Autodesk Fusion 360 part; units mm, degrees
note: some values were not read from the file. Set by a fixed rule: which sketch regions a step uses.
(part 4 of 4)
sketch "Sketch12" plane through (0, 0, 0) normal (0, 0, -1) x (1, 0, 0)
  arc A0 (214.104, -171.958) -> (214.104, -165.862) centre (214.104, -168.91) ccw
  line L0 (214.104, -171.958) -> (197.3761, -171.958)
  arc A1 (197.3761, -165.862) -> (197.3761, -171.958) centre (197.3761, -168.91) ccw
  line L1 (197.3761, -165.862) -> (214.104, -165.862)
  arc A2 (216.662, -132.8241) -> (222.758, -132.8241) centre (219.71, -132.8241) ccw
  line L2 (216.662, -132.8241) -> (216.662, -113.5562)
  arc A3 (222.758, -113.5562) -> (216.662, -113.5562) centre (219.71, -113.5562) ccw
  line L3 (222.758, -113.5562) -> (222.758, -132.8241)
  arc A4 (247.142, -132.8241) -> (253.238, -132.8241) centre (250.19, -132.8241) ccw
  line L4 (247.142, -132.8241) -> (247.142, -113.5562)
  arc A5 (253.238, -113.5562) -> (247.142, -113.5562) centre (250.19, -113.5562) ccw
  line L5 (253.238, -113.5562) -> (253.238, -132.8241)
  arc A6 (253.238, -144.0361) -> (247.142, -144.0361) centre (250.19, -144.0361) ccw
  line L6 (253.238, -144.0361) -> (253.238, -163.304)
  arc A7 (247.142, -163.304) -> (253.238, -163.304) centre (250.19, -163.304) ccw
  line L7 (247.142, -163.304) -> (247.142, -144.0361)
  line L8 (275.082, -163.304) -> (275.082, -144.0361)
  arc A8 (281.178, -144.0361) -> (275.082, -144.0361) centre (278.13, -144.0361) ccw
  line L9 (281.178, -144.0361) -> (281.178, -163.304)
  arc A9 (275.082, -163.304) -> (281.178, -163.304) centre (278.13, -163.304) ccw
  arc A10 (255.796, -104.9022) -> (255.796, -110.9982) centre (255.796, -107.9502) ccw
  line L10 (255.796, -104.9022) -> (272.5239, -104.9022)
  arc A11 (272.5239, -110.9982) -> (272.5239, -104.9022) centre (272.5239, -107.9502) ccw
  line L11 (272.5239, -110.9982) -> (255.796, -110.9982)
  arc A12 (188.722, -132.824) -> (194.818, -132.8241) centre (191.77, -132.824) ccw
  line L12 (188.722, -132.824) -> (188.722, -113.5562)
  arc A13 (194.818, -113.5562) -> (188.722, -113.5562) centre (191.77, -113.5562) ccw
  line L13 (194.818, -113.5562) -> (194.818, -132.8241)
  arc A14 (194.818, -144.0361) -> (188.722, -144.0361) centre (191.77, -144.0361) ccw
  line L14 (194.818, -144.0361) -> (194.818, -163.304)
  arc A15 (188.722, -163.304) -> (194.818, -163.304) centre (191.77, -163.304) ccw
  line L15 (188.722, -163.304) -> (188.722, -144.0361)
  arc A16 (214.104, -141.4781) -> (214.104, -135.3821) centre (214.104, -138.4301) ccw
  line L16 (214.104, -141.4781) -> (197.3761, -141.4781)
  arc A17 (197.3761, -135.3821) -> (197.3761, -141.4781) centre (197.3761, -138.4301) ccw
  line L17 (197.3761, -135.3821) -> (214.104, -135.3821)
  circle A18 centre (234.95, -107.95) radius 2.921
  arc A19 (255.796, -135.3821) -> (255.796, -141.4781) centre (255.796, -138.4301) ccw
  line L18 (255.796, -135.3821) -> (272.5239, -135.3821)
  arc A20 (272.5239, -141.4781) -> (272.5239, -135.3821) centre (272.5239, -138.4301) ccw
  line L19 (272.5239, -141.4781) -> (255.796, -141.4781)
  arc A21 (255.796, -165.862) -> (255.796, -171.958) centre (255.796, -168.91) ccw
  line L20 (255.796, -165.862) -> (272.5239, -165.862)
  arc A22 (272.5239, -171.958) -> (272.5239, -165.862) centre (272.5239, -168.91) ccw
  line L21 (272.5239, -171.958) -> (255.796, -171.958)
  arc A23 (275.082, -132.8241) -> (281.178, -132.824) centre (278.13, -132.824) ccw
  line L22 (275.082, -132.8241) -> (275.082, -113.5562)
  arc A24 (281.178, -113.5562) -> (275.082, -113.5562) centre (278.13, -113.5562) ccw
  line L23 (281.178, -113.5562) -> (281.178, -132.824)
  arc A25 (214.104, -110.9982) -> (214.104, -104.9022) centre (214.104, -107.9502) ccw
  line L24 (214.104, -110.9982) -> (197.3761, -110.9982)
  arc A26 (197.3761, -104.9022) -> (197.3761, -110.9982) centre (197.3761, -107.9502) ccw
  line L25 (197.3761, -104.9022) -> (214.104, -104.9022)
  arc A27 (222.758, -144.0361) -> (216.662, -144.0361) centre (219.71, -144.0361) ccw
  line L26 (222.758, -144.0361) -> (222.758, -163.304)
  arc A28 (216.662, -163.304) -> (222.758, -163.304) centre (219.71, -163.304) ccw
  line L27 (216.662, -163.304) -> (216.662, -144.0361)
  line L28 (297.18, -102.87) -> (172.72, -102.87)
  line L29 (172.72, -102.87) -> (172.72, -189.23)
  line L30 (172.72, -189.23) -> (297.18, -189.23)
  line L31 (297.18, -189.23) -> (297.18, -102.87)
  circle A29 centre (281.94, -180.34) radius 1.5875
  circle A30 centre (189.23, -180.34) radius 1.5875
  circle A31 centre (189.23, -110.49) radius 1.5875
  circle A32 centre (281.94, -110.49) radius 1.5875
  circle A33 centre (281.94, -180.34) radius 5.08
  circle A34 centre (281.94, -180.34) radius 2.2225
  circle A35 centre (189.23, -180.34) radius 2.2225
  circle A36 centre (189.23, -180.34) radius 5.08
  circle A37 centre (281.94, -110.49) radius 5.08
  circle A38 centre (281.94, -110.49) radius 2.2225
  circle A39 centre (189.23, -110.49) radius 2.2225
  circle A40 centre (189.23, -110.49) radius 5.08
  line L32 (297.18, -189.23) -> (294.64, -189.23)
  line L33 (294.64, -189.23) -> (294.64, -187.96)
  line L34 (294.64, -187.96) -> (297.18, -187.96)
  line L35 (297.18, -187.96) -> (297.18, -189.23)
  line L36 (172.72, -102.87) -> (175.26, -102.87)
  line L37 (175.26, -102.87) -> (175.26, -104.14)
  line L38 (175.26, -104.14) -> (172.72, -104.14)
  line L39 (172.72, -104.14) -> (172.72, -102.87)
  line L40 (294.64, -187.96) -> (175.26, -187.96)
  line L41 (175.26, -187.96) -> (175.26, -104.14)
  line L42 (175.26, -104.14) -> (294.64, -104.14)
  line L43 (294.64, -104.14) -> (294.64, -187.96)
  point P0 (281.94, -180.34)
  point P1 (189.23, -180.34)
  point P2 (189.23, -110.49)
  point P3 (281.94, -110.49)
  dimension "d121" = 10.16
  dimension "d122" = 4.445
  dimension "d123" = 4.445
  dimension "d124" = 10.16
  dimension "d125" = 10.16
  dimension "d126" = 4.445
  dimension "d127" = 4.445
  dimension "d128" = 10.16
  dimension "d129" = 2.54
  dimension "d130" = 1.27
  dimension "d131" = 2.54
  dimension "d132" = 1.27
  constraint coincident P0 A29.centre
  constraint coincident P1 A30.centre
  constraint coincident P2 A31.centre
  constraint coincident P3 A32.centre
  constraint concentric A29 A33
  constraint concentric A30 A35
  constraint concentric A32 A37
  constraint concentric A32 A38
  constraint horizontal L32
  constraint vertical L33
  constraint horizontal L34
  constraint vertical L35
  constraint coincident L30.end L31.start
  constraint horizontal L36
  constraint vertical L37
  constraint horizontal L38
  constraint vertical L39
  constraint coincident L28.end L29.start
  constraint horizontal L40
  constraint vertical L41
  constraint horizontal L42
  constraint vertical L43
  measures "d121" diameter of A33
  measures "d122" diameter of A34
  measures "d123" diameter of A35
  measures "d124" diameter of A36
  measures "d125" diameter of A37
  measures "d126" diameter of A38
  measures "d127" diameter of A39
  measures "d128" diameter of A40
  measures "d129" distance of L30.end L32.end
  measures "d130" distance of L30.end L34.end
  measures "d131" distance of L28.end L36.end
  measures "d132" distance of L28.end L38.end
extrude "Extrude22" cut sketch "Sketch12" against normal blind 5.08 contours L40 L41 L42 L43 bodies 1
extrude "Extrude23" cut sketch "Sketch12" against normal blind 12.7 contours A13 A31 A39 | A13 A31 | A24 A38 | A29 | A30 | A32 | A34 | A35 picked at (191.1543, -110.3249) picked at (189.3012, -110.5595) picked at (280.0788, -110.98) bodies 1
extrude "Extrude24" cut 4 faces at (280.7797, 184.2894, 0) (188.6713, 184.4182, 0) (187.7629, 113.5699, 0) (278.5579, 109.5942, 0) along direction (0, 0, 1) blind 2.54 on bodies 1 bodies 1
sketch "Sketch13" plane through (297.18, 0, 0) normal (1, 0, 0) x (0, 1, 0)
  line L0 (189.23, 19.05) -> (102.87, 19.05)
  line L1 (102.87, 19.05) -> (102.87, 0)
  line L2 (102.87, 0) -> (189.23, 0)
  line L3 (189.23, 0) -> (189.23, 19.05)
  line L4 (189.23, 0) -> (173.99, 0)
  line L5 (173.99, 0) -> (173.99, 5.08)
  line L6 (173.99, 5.08) -> (189.23, 5.08)
  line L7 (189.23, 5.08) -> (189.23, 0)
  line L8 (102.87, 0) -> (118.11, 0)
  line L9 (118.11, 0) -> (118.11, 5.08)
  line L10 (118.11, 5.08) -> (102.87, 5.08)
  line L11 (102.87, 5.08) -> (102.87, 0)
  dimension "d139" = 15.24
  dimension "d140" = 5.08
  dimension "d141" = 15.24
  dimension "d142" = 5.08
  constraint horizontal L4
  constraint vertical L5
  constraint horizontal L6
  constraint vertical L7
  constraint coincident L2.end L3.start
  constraint horizontal L8
  constraint vertical L9
  constraint horizontal L10
  constraint vertical L11
  constraint coincident L1.end L2.start
  measures "d139" distance of L2.end L4.end
  measures "d140" distance of L2.end L6.end
  measures "d141" distance of L1.end L8.end
  measures "d142" distance of L1.end L10.end
extrude "Extrude25" add sketch "Sketch13" along normal blind 15.24 contours L2 L3 L4 L5 L6 L7 | L1 L2 L8 L9 L10 L11 bodies 1
sketch "Sketch14" plane through (0, 0, 5.08) normal (0, 0, 1) x (-1, 0, 0)
  line L0 (-297.18, -189.23) -> (-297.18, -173.99)
  line L1 (-297.18, -173.99) -> (-312.42, -173.99)
  line L2 (-312.42, -173.99) -> (-312.42, -189.23)
  line L3 (-312.42, -189.23) -> (-297.18, -189.23)
  circle A0 centre (-304.8, -181.61) radius 2.286
  circle A1 centre (-304.8, -110.49) radius 2.286
  dimension "d145" = 4.572
  dimension "d146" = 4.572
  measures "d145" diameter of A0
  measures "d146" diameter of A1
extrude "Extrude26" cut sketch "Sketch14" against normal blind 25.4 contours A0 | A1 bodies 1
chamfer "Chamfer1" distance 4.064 angle 45 2 edges at (306.9313, 111.3167, 0) (306.9313, 182.4367, 0) on bodies 1
sketch "Sketch15" plane through (172.72, 0, 0) normal (-1, 0, 0) x (0, -1, 0)
  line L0 (-102.87, 19.05) -> (-189.23, 19.05)
  line L1 (-189.23, 19.05) -> (-189.23, 0)
  line L2 (-189.23, 0) -> (-102.87, 0)
  line L3 (-102.87, 0) -> (-102.87, 19.05)
  line L4 (-102.87, 0) -> (-118.11, 0)
  line L5 (-118.11, 0) -> (-118.11, 5.08)
  line L6 (-118.11, 5.08) -> (-102.87, 5.08)
  line L7 (-102.87, 5.08) -> (-102.87, 0)
  line L8 (-189.23, 0) -> (-173.99, 0)
  line L9 (-173.99, 0) -> (-173.99, 5.08)
  line L10 (-173.99, 5.08) -> (-189.23, 5.08)
  line L11 (-189.23, 5.08) -> (-189.23, 0)
  dimension "d150" = 15.24
  dimension "d151" = 5.08
  dimension "d152" = 15.24
  dimension "d153" = 5.08
  constraint horizontal L4
  constraint vertical L5
  constraint horizontal L6
  constraint vertical L7
  constraint coincident L2.end L3.start
  constraint horizontal L8
  constraint vertical L9
  constraint horizontal L10
  constraint vertical L11
  constraint coincident L1.end L2.start
  measures "d150" distance of L2.end L4.end
  measures "d151" distance of L2.end L6.end
  measures "d152" distance of L1.end L8.end
  measures "d153" distance of L1.end L10.end
extrude "Extrude27" add sketch "Sketch15" along normal blind 15.24 contours L2 L3 L4 L5 L6 L7 | L1 L2 L8 L9 L10 L11 bodies 1
sketch "Sketch16" plane through (0, 0, 5.08) normal (0, 0, 1) x (-1, 0, 0)
  line L0 (-172.72, -102.87) -> (-172.72, -118.11)
  line L1 (-172.72, -118.11) -> (-157.48, -118.11)
  line L2 (-157.48, -118.11) -> (-157.48, -102.87)
  line L3 (-157.48, -102.87) -> (-172.72, -102.87)
  circle A0 centre (-165.1, -110.49) radius 2.286
  circle A1 centre (-165.1, -181.61) radius 2.286
  dimension "d156" = 4.572
  dimension "d157" = 4.572
  measures "d156" diameter of A0
  measures "d157" diameter of A1
extrude "Extrude28" cut sketch "Sketch16" against normal blind 25.4 contours A0 | A1 bodies 1
chamfer "Chamfer2" distance 4.064 angle 45 2 edges at (167.2313, 111.3167, 0) (167.2313, 182.4367, 0) on bodies 1
fillet "Fillet1" radius 5.08 2 edges at (157.48, 102.87, 2.54) (157.48, 118.11, 2.54) on bodies 1
fillet "Fillet2" radius 5.08 6 edges at (157.48, 173.99, 2.54) (157.48, 189.23, 2.54) (312.42, 102.87, 2.54) (312.42, 118.11, 2.54) (312.42, 189.23, 2.54) (312.42, 173.99, 2.54) on bodies 1
fillet "Fillet3" radius 5.08 4 edges at (297.18, 102.87, 12.065) (297.18, 189.23, 12.065) (172.72, 189.23, 12.065) (172.72, 102.87, 12.065) on bodies 1
sketch "Sketch17" plane through (0, 0, 0) normal (0, 0, 1) x (1, 0, 0)
sketch "Sketch18" plane through (0, 0, 0) normal (0, 0, 1) x (1, 0, 0)
  line L0 (-25.4, 0) -> (-50.8, 0)
  line L1 (-50.8, 0) -> (-50.8, 25.4)
  line L2 (-50.8, 25.4) -> (-25.4, 25.4)
  line L3 (-25.4, 25.4) -> (-25.4, 0)
  circle A0 centre (-38.1, 12.7) radius 3.175
  dimension "d167" = 25.4
  dimension "d168" = 6.35
  constraint horizontal L0
  constraint vertical L1
  constraint horizontal L2
  constraint vertical L3
  measures "d167" distance of L0.start L0.end
  measures "d168" diameter of A0
